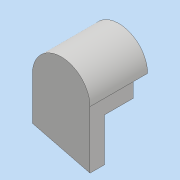
# Autodesk Inventor part: 6
Saved by Autodesk Inventor 2017 (Build 210142000, 142)
## iProperties
Part Number: 6
Material: 一般
Document SubType Name: Modeling
Designer: d8910
Density: 1 g/cm^3
Appearance: 預設
Author: d8910
Autodesk Inventor part; units mm, degrees
ref_plane "YZ Plane" through (0, 0, 0) normal (1, 0, 0) x (0, 1, 0)
ref_plane "XZ Plane" through (0, 0, 0) normal (0, 1, 0) x (-1, 0, 0)
ref_plane "XY Plane" through (0, 0, 0) normal (0, 0, 1) x (1, 0, 0)
sketch "草圖1" plane through (0, 0, 0) normal (0, 1, 0) x (-1, 0, 0)
  line L0 (-10, 5) -> (-10, -15)
  line L1 (10, -10) -> (10, 5)
  arc A0 (10, 5) -> (-10, 5) centre (0, 5) ccw
  line L2 (-10, -15) -> (10, -10)
  point P0 (0, 0)
  point P1 (0, -10)
  point P2 (10, 0)
  dimension "d0" = 20
  dimension "d1" = 20
  dimension "d2" = 15
  dimension "d3" = 10
  dimension "d4" = 10
  constraints: 6 end point, 2 point on circle, 2 tangent, 2 vertical alignment, 1 centre point, 1 horizontal alignment, 1 parallel, 1 point on line
  measures "d0" distance of L0.start L0.end
  measures "d1" distance between parallel lines of L0 L1
  measures "d2" distance of L1.start L1.end
  measures "d3" horizontal distance of L1.start point (0, 0)
  measures "d4" distance from line of point (0, 0) L0
extrude "擠出1" add sketch "草圖1" along normal blind 5
sketch "草圖2" plane through (0, 5, 0) normal (0, 1, 0) x (1, 0, 0)
  line L0 (-10, 10) -> (-10, -5) construction
  arc A0 (-10, -5) -> (10, -5) centre (0, -5) ccw projected
  line L1 (10, -5) -> (10, 15) construction
  line L2 (10, 15) -> (-10, 10) construction
  arc A1 (-10, -5) -> (10, -5) centre (0, -5) ccw projected
  line L3 (10, -5) -> (10, 0)
  line L4 (10, 0) -> (-10, 5)
  line L5 (-10, 10) -> (-10, -5) projected
  line L6 (-10, -5) -> (-10, 5)
  point P0 (0, 0)
  dimension "d7" = 5
  dimension "d8" = 15
  constraints: 6 end point, 2 point on line, 2 tangent, 1 parallel
  measures "d7" distance of L0.start L4.end
  measures "d8" distance of L1.end L3.end
extrude "擠出2" add sketch "草圖2" along normal blind 10
sketch "草圖3" plane through (0, 15, 0) normal (0, 1, 0) x (1, 0, 0)
  arc A0 (-10, -5) -> (10, -5) centre (0, -5) ccw projected
  line L0 (10, -5) -> (10, 0) construction
  line L1 (10, 0) -> (-10, 5) construction
  line L2 (-10, 5) -> (-10, -5) construction
  line L3 (10, -5) -> (-10, 0)
  line L4 (-10, -5) -> (-10, 10) projected
  line L5 (-10, -5) -> (-10, 0)
  point P0 (0, 0)
  dimension "d11" = 5
  constraints: 4 end point, 1 collinear, 1 point on line
  measures "d11" distance of L3.end L2.end
extrude "擠出3" add sketch "草圖3" along normal blind 5
